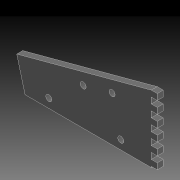
# Autodesk Inventor part: KB33-046-004-009 - Передняя левая боковая пластина
Saved by Autodesk Inventor 2020 (Build 240168000, 168)
## iProperties
Created: 2021-06-25
Part Number: KB33-046-004-009 - Передняя левая боковая пластина
Material: Типовые
Document SubType Name: Modeling
Designer: Петров Иван
Mass: 11.6787 g
Surface Area: 72.0455 cm^2
Volume: 11.6787 cm^3
Density: 1 g/cm^3
Appearance: По умолчанию
Author: Петров Иван
Autodesk Inventor part; units mm, degrees
ref_plane "YZ Plane" through (0, 0, 0) normal (1, 0, 0) x (0, 1, 0)
ref_plane "XZ Plane" through (0, 0, 0) normal (0, 1, 0) x (-1, 0, 0)
ref_plane "XY Plane" through (0, 0, 0) normal (0, 0, 1) x (1, 0, 0)
sketch "Эскиз1" plane through (0, 0, 0) normal (0, 0, 1) x (1, 0, 0)
  line L0 (-1.0718, 4) -> (83.0251, 4)
  circle A0 centre (14.7479, 10) radius 2
  circle A1 centre (62.7479, 10) radius 2
  line L1 (-1.0718, 4) -> (-3.896, 14.54)
  line L2 (83.0251, 4) -> (83.0251, 48.71)
  line L3 (-3.896, 14.54) -> (-6.6159, 24.6909)
  line L4 (-6.6159, 24.6909) -> (83.0251, 48.71)
  dimension "d0" = 10.509
  constraints: 10 end point, 2 centre point, 1 point on line
  measures "d0" distance of L1.end L3.end
extrude "Выдавливание1" add sketch "Эскиз1" along normal blind 4
sketch "Эскиз2" plane through (83.0251, 4, 0) normal (1, 0, 0) x (0, 0, -1)
  line L0 (-4, 0) -> (-4, 44.71) projected
  line L1 (0, 0) -> (0, 44.71) projected
  line L2 (-4, 44.71) -> (0, 44.71)
  line L3 (0, 44.71) -> (0, 40.71)
  line L4 (0, 40.71) -> (-4, 40.71)
  line L5 (-4, 40.71) -> (-4, 44.71)
  point P0 (0, -4)
  point P1 (-4, 40.71)
  dimension "d3" = 4
  constraints: 8 end point, 2 parallel, 1 horizontal, 1 perpendicular, 1 point on line
  measures "d3" distance of L2.end L3.end
extrude "Выдавливание2" add sketch "Эскиз2" along normal blind 4
pattern_linear "Прямоуг.массив1" count 6 spacing 8 along (0, -1, 0) of "Выдавливание2"
sketch "Эскиз3" plane through (0, 0, 4) normal (0, 0, 1) x (1, 0, 0)
  circle A0 centre (56.9359, 33.9549) radius 2 projected
  line L0 (-6.6159, 24.6909) -> (-1.0718, 4) projected
  line L1 (-1.0718, 4) -> (83.0251, 4) projected
  line L2 (83.0251, 4) -> (83.0251, 4.71) projected
  line L3 (83.0251, 4.71) -> (87.0251, 4.71) projected
  line L4 (87.0251, 8.71) -> (87.0251, 4.71) projected
  line L5 (83.0251, 8.71) -> (87.0251, 8.71) projected
  line L6 (83.0251, 8.71) -> (83.0251, 12.71) projected
  line L7 (83.0251, 12.71) -> (87.0251, 12.71) projected
  line L8 (87.0251, 16.71) -> (87.0251, 12.71) projected
  line L9 (83.0251, 16.71) -> (87.0251, 16.71) projected
  line L10 (83.0251, 16.71) -> (83.0251, 20.71) projected
  line L11 (83.0251, 20.71) -> (87.0251, 20.71) projected
  line L12 (87.0251, 24.71) -> (87.0251, 20.71) projected
  line L13 (83.0251, 24.71) -> (87.0251, 24.71) projected
  line L14 (83.0251, 24.71) -> (83.0251, 28.71) projected
  line L15 (83.0251, 28.71) -> (87.0251, 28.71) projected
  line L16 (87.0251, 32.71) -> (87.0251, 28.71) projected
  line L17 (83.0251, 32.71) -> (87.0251, 32.71) projected
  line L18 (83.0251, 32.71) -> (83.0251, 36.71) projected
  line L19 (83.0251, 36.71) -> (87.0251, 36.71) projected
  line L20 (87.0251, 40.71) -> (87.0251, 36.71) projected
  line L21 (83.0251, 40.71) -> (87.0251, 40.71) projected
  line L22 (83.0251, 40.71) -> (83.0251, 44.71) projected
  line L23 (83.0251, 44.71) -> (87.0251, 44.71) projected
  line L24 (87.0251, 48.71) -> (87.0251, 44.71) projected
  line L25 (83.0251, 48.71) -> (87.0251, 48.71) projected
  line L26 (83.0251, 48.71) -> (-6.6159, 24.6909) projected
  circle A1 centre (62.7479, 10) radius 2 projected
  circle A2 centre (14.7479, 10) radius 2 projected
  circle A3 centre (37.6174, 28.7785) radius 2 projected
  point P0 (0, 0)
extrude "Выдавливание3" cut sketch "Эскиз3" against normal blind 10 contours A0 | A3
